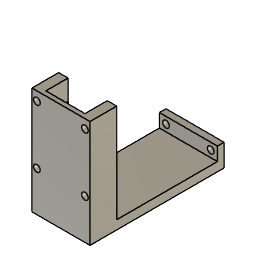
Potentiometer L-bracket (Autodesk Fusion 360 design; units mm, degrees)
Autodesk Fusion 360 part; units mm, degrees
sketch "Sketch1" plane through (0, 0, 0) normal (0, 0, 1) x (1, 0, 0)
  line L0 (0, 0) -> (26, 0)
  line L1 (26, 0) -> (26, 60)
  line L2 (26, 60) -> (0, 60)
  line L3 (0, 60) -> (0, 0)
  line L4 (0, 0) -> (26, 0)
  line L5 (26, 0) -> (26, 12)
  line L6 (26, 12) -> (0, 12)
  line L7 (0, 12) -> (0, 0)
  line L8 (0, 60) -> (26, 60)
  line L9 (26, 60) -> (26, 57)
  line L10 (26, 57) -> (0, 57)
  line L11 (0, 57) -> (0, 60)
  dimension "d1" = 26
  dimension "d2" = 60
  dimension "d16" = 48
  dimension "d43" = 3
  constraint horizontal L0
  constraint vertical L1
  constraint horizontal L2
  constraint vertical L3
  constraint coincident L0.start L3.end
  constraint horizontal L4
  constraint vertical L5
  constraint horizontal L6
  constraint vertical L7
  constraint coincident L1 L5.end
  constraint horizontal L8
  constraint vertical L9
  constraint horizontal L10
  constraint vertical L11
  measures "d1" distance of L1 L3
  measures "d2" distance of L0 L2
  measures "d16" distance of L2 L6
  measures "d43" distance of L2 L10
extrude "Extrude1" add sketch "Sketch1" along normal blind 4 contours L1 L3 L6 L10
extrude "Extrude2" add sketch "Sketch1" along normal blind 48 contours L0 L1 L3 L4 L5 L6 L7
extrude "Extrude6" add sketch "Sketch1" along normal blind 10 contours L1 L2 L3 L8 L9 L10 L11
sketch "Sketch2" plane through (0, 12, 0) normal (0, 1, 0) x (-1, 0, 0)
  line L0 (-26, 4) -> (0, 4)
  line L1 (0, 4) -> (0, 48)
  line L2 (0, 48) -> (-26, 48)
  line L3 (-26, 48) -> (-26, 4)
  circle A0 centre (-13, 39) radius 8.75
  line L4 (-21.75, 39) -> (-21.75, 48)
  line L5 (-4.25, 39) -> (-4.25, 48)
  dimension "d17" = 17.5
  dimension "d27" = 13
  dimension "d28" = 4.25
  dimension "d46" = 35
  constraint coincident A0 L4.start
  constraint coincident L2 L4.end
  constraint perpendicular L2 L4
  constraint coincident A0 L5.start
  constraint tangent A0 L5
  constraint coincident L2 L5.end
  constraint perpendicular L2 L5
  measures "d17" diameter of A0
  measures "d27" distance of L1 A0.centre
  measures "d28" distance of L3 L4
  measures "d46" distance of L0 A0.centre
extrude "Extrude3" cut sketch "Sketch2" against normal blind 10 contours L2 A0 L4 L5 | A0
sketch "Sketch3" plane through (0, 12, 0) normal (0, 1, 0) x (-1, 0, 0)
  line L0 (-26, 4) -> (0, 4)
  line L1 (0, 4) -> (0, 48)
  line L2 (-21.75, 48) -> (-26, 48)
  line L3 (-26, 48) -> (-26, 4)
  line L4 (-21.75, 39) -> (-21.75, 48)
  line L5 (0, 48) -> (-4.25, 48)
  line L6 (-4.25, 48) -> (-4.25, 39)
  arc A0 (-21.75, 39) -> (-4.25, 39) centre (-13, 39) ccw
  circle A1 centre (-23.75, 44) radius 1.5
  circle A2 centre (-2.25, 44) radius 1.5
  circle A3 centre (-23.75, 18) radius 1.5
  circle A4 centre (-2.25, 18) radius 1.5
  dimension "d29" = 3
  dimension "d30" = 2.25
  dimension "d31" = 3
  dimension "d32" = 2.25
  dimension "d33" = 3
  dimension "d34" = 3
  dimension "d35" = 2.25
  dimension "d36" = 2.25
  dimension "d37" = 4
  dimension "d38" = 4
  dimension "d57" = 30
  dimension "d58" = 30
  measures "d29" diameter of A1
  measures "d30" distance of L3 A1.centre
  measures "d31" diameter of A2
  measures "d32" distance of L1 A2.centre
  measures "d33" diameter of A3
  measures "d34" diameter of A4
  measures "d35" distance of L3 A3.centre
  measures "d36" distance of L1 A4.centre
  measures "d37" distance of L5 A2.centre
  measures "d38" distance of L2 A1.centre
  measures "d57" distance of L2 A3.centre
  measures "d58" distance of L5 A4.centre
extrude "Extrude5" cut sketch "Sketch3" against normal blind 13 contours A1 | A2 | A3 | A4
sketch "Sketch4" plane through (0, 60, 0) normal (0, 1, 0) x (-1, 0, 0)
  line L0 (-26, 0) -> (0, 0)
  line L1 (0, 0) -> (0, 10)
  line L2 (0, 10) -> (-26, 10)
  line L3 (-26, 10) -> (-26, 0)
  circle A0 centre (-3, 7) radius 1.5
  circle A1 centre (-23, 7) radius 1.5
  dimension "d49" = 3
  dimension "d50" = 3
  dimension "d51" = 3
  dimension "d52" = 3
  dimension "d53" = 3
  dimension "d54" = 3
  measures "d49" diameter of A0
  measures "d50" diameter of A1
  measures "d51" distance of L1 A0.centre
  measures "d52" distance of L2 A0.centre
  measures "d53" distance of L2 A1.centre
  measures "d54" distance of L3 A1.centre
extrude "Extrude7" cut sketch "Sketch4" against normal blind 4 contours A0 | A1
